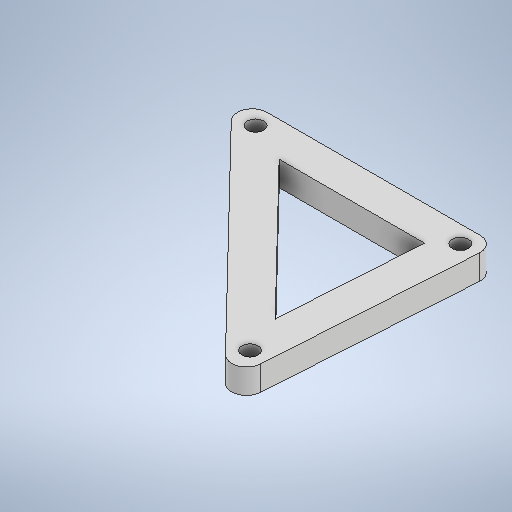
# Autodesk Inventor part: bde
Saved by Autodesk Inventor 2025.1 (Build 291241020, 241B)
## iProperties
Created: 2025-05-24
Part Number: bde
Material: Generic
Document SubType Name: Modeling
Designer: omiye
Density: 1 g/cm^3
Appearance: Default
Author: omiye
Autodesk Inventor part; units mm, degrees
ref_plane "YZ Plane" through (0, 0, 0) normal (1, 0, 0) x (0, 1, 0)
ref_plane "XZ Plane" through (0, 0, 0) normal (0, 1, 0) x (-1, 0, 0)
ref_plane "XY Plane" through (0, 0, 0) normal (0, 0, 1) x (1, 0, 0)
sketch "Sketch1" plane through (0, 0, 0) normal (0, 1, 0) x (-1, 0, 0)
  line L0 (0, 0) -> (41.5, 0)
  line L1 (41.5, 0) -> (2.6101, 40.0152)
  line L2 (2.6101, 40.0152) -> (0, 0)
  line L3 (-38.7898, 77.591) -> (-33.77, 82.4696)
  line L4 (-33.77, 82.4696) -> (44.0099, 2.4393)
  line L5 (44.0099, 2.4393) -> (38.9901, -2.4393)
  line L6 (38.9901, -2.4393) -> (-38.7898, 77.591)
  line L7 (-38.7898, 77.591) -> (44.0099, 2.4393) construction
  line L8 (-33.77, 82.4696) -> (38.9901, -2.4393) construction
  line L9 (83, -3.5) -> (83, 3.5)
  line L10 (83, 3.5) -> (0, 3.5)
  line L11 (0, 3.5) -> (0, -3.5)
  line L12 (0, -3.5) -> (83, -3.5)
  line L13 (83, -3.5) -> (0, 3.5) construction
  line L14 (83, 3.5) -> (0, -3.5) construction
  line L15 (-6.1026, -39.7873) -> (0.8825, -40.243)
  line L16 (0.8825, -40.243) -> (6.1026, 39.7873)
  line L17 (6.1026, 39.7873) -> (-0.8825, 40.243)
  line L18 (-0.8825, 40.243) -> (-6.1026, -39.7873)
  line L19 (-6.1026, -39.7873) -> (6.1026, 39.7873) construction
  line L20 (0.8825, -40.243) -> (-0.8825, 40.243) construction
  circle A0 centre (0, 0) radius 1.65
  circle A1 centre (2.6101, 40.0152) radius 1.65
  circle A2 centre (41.5, 0) radius 1.65
  line L21 (2.6101, 40.0152) -> (-2.6009, 40.355)
  line L22 (-1.2742, 34.2377) -> (-0.3698, 48.1031)
  line L23 (-0.3698, 48.1031) -> (-5.0836, 42.9096)
  line L24 (-2.6009, 40.355) -> (2.1129, 45.5486)
  line L25 (6.5967, -3.5) -> (-3.7357, -3.5)
  line L26 (10.4211, 3.5) -> (-3.2791, 3.5)
  line L27 (44.9726, 3.5) -> (44.9726, -3.5731)
  point P0 (33.2178, 3.5)
  point P1 (3.7357, 3.5)
  point P2 (5.5899, 31.9272)
  point P3 (42.9791, 3.5)
  point P4 (-0.7416, 42.4036)
  point P5 (44.9726, -3.5)
  dimension "d0" = 41.5
  dimension "d1" = 55.8
  dimension "d2" = 45.817
  dimension "d3" = 7
  dimension "d4" = 7
  dimension "d5" = 7
  dimension "d6" = 3.3
  dimension "d7" = 3.3
  dimension "d8" = 3.3
  constraints: 56 end point, 14 point on line, 7 parallel, 6 midpoint, 5 perpendicular, 3 centre point, 3 coincident, 1 horizontal, 1 vertical
  measures "d0" distance of L0.start L0.end
  measures "d1" distance of L0.end L1.end
  measures "d2" angle of L1 L0
  measures "d3" distance of L3.start L3.end
  measures "d4" distance of L9.start L9.end
  measures "d5" distance of L15.start L15.end
  measures "d6" diameter of A0
  measures "d7" diameter of A1
  measures "d8" diameter of A2
extrude "Extrusion1" add sketch "Sketch1" along normal blind 5 contours A0 L2 L10 L16 L0 | L0 L16 L12 L11 A0 | A0 L11 L10 L2 | A0 L11 L25 L18 L26 | L16 L10 L6 L0 | L0 L6 L5 A2 L4 L10 L27 L12 L16 | L10 L26 L18 L6 L2 | L2 L6 L16 L10 | L6 L10 L1 A2 L0 | L0 A2 L5 L6 | L6 L18 L17 A1 L2 | L2 A1 L1 L16 L6 | L6 L16 L1 L10 | L1 L10 L4 L5 A2 | L1 L16 L17 A1 L22 L24 L4 L10 | L1 A1 L17 L16
sketch "Sketch2" plane through (0, 5, 0) normal (0, 1, 0) x (1, 0, 0)
  line L0 (-42.9791, -3.5) -> (-2.1129, -45.5486) projected
  line L1 (-41.9322, -4.5771) -> (-44.9726, -1.4485)
  line L2 (-44.9726, 3.5) -> (-44.9726, -3.5) projected
  line L3 (-41.9322, -4.5771) -> (-37.5696, -4.5771) construction
  line L4 (-44.9726, -1.4485) -> (-44.9726, -3.5)
  line L5 (-44.9726, -3.5) -> (-42.9791, -3.5)
  point P0 (0, 0)
  dimension "d11" = 134.18
  constraints: 8 end point, 2 point on line, 1 collinear, 1 equal length, 1 horizontal, 1 perpendicular
  measures "d11" angle of L3 L1
extrude "Extrusion2" cut sketch "Sketch2" against normal blind 10
sketch "Sketch3" plane through (0, 5, 0) normal (0, 1, 0) x (1, 0, 0)
  line L0 (-44.9726, -1.4485) -> (-41.9322, -4.5771) projected
  line L1 (-44.9726, 3.5) -> (-44.9726, -1.4485)
  line L2 (-44.9726, -1.4485) -> (-44.9726, 3.5)
  line L3 (-44.9726, 3.5) -> (-53.5355, 3.5)
  line L4 (-41.9322, -4.5771) -> (-49.7814, 3.5)
  line L5 (-41.9322, -4.5771) -> (-2.1129, -45.5486) projected
  line L6 (-6.7195, -40.8087) -> (1.7936, -49.5681)
  line L7 (0.7416, -42.4036) -> (3.7357, 3.5) projected
  line L8 (0.9497, -39.2136) -> (0.3698, -48.1031)
  line L9 (-2.1129, -45.5486) -> (0.7416, -42.4036) projected
  line L10 (-2.1129, -45.5486) -> (0.7416, -42.4036)
  point P0 (0, 0)
  constraints: 14 end point, 4 collinear, 3 point on line, 1 horizontal, 1 vertical
extrude "Extrusion3" add sketch "Sketch3" against normal blind 5
fillet "Fillet1" radius 3 3 edges at (0.3698, 2.5, 48.1031) (-49.7814, 2.5, -3.5) (3.7357, 2.5, -3.5)
body "Solid1"
